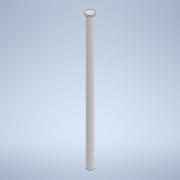
# Autodesk Inventor part: q1
Saved by Autodesk Inventor 2022 (Build 260153000, 153)
## iProperties
Created: 2023-05-29
Part Number: q1
Material: Ogólny
Document SubType Name: Modeling
Designer: nosal
Density: 1 g/cm^3
Appearance: Domyślna
Author: nosal
## iProperties of the stored document q1_Drukowanie 3D.ipt
Created: 2023-05-29
Part Number: q1_Drukowanie 3D
Material: Ogólny
Document SubType Name: Modeling
Designer: nosal
Density: 1 g/cm^3
Appearance: Domyślna
Author: nosal
Autodesk Inventor part; units mm, degrees
ref_plane "YZ Plane" through (0, 0, 0) normal (1, 0, 0) x (0, 1, 0)
ref_plane "XZ Plane" through (0, 0, 0) normal (0, 1, 0) x (-1, 0, 0)
ref_plane "XY Plane" through (0, 0, 0) normal (0, 0, 1) x (1, 0, 0)
sketch "Szkic1" plane through (0, 0, 0) normal (0, 0, 1) x (1, 0, 0)
  line L0 (0, 0) -> (-4, 0)
  line L1 (-4, 0) -> (-4, 175)
  line L2 (-4, 175) -> (0, 175)
  line L3 (0, 175) -> (0, 0)
  line L4 (-4, 175) -> (-5, 175)
  line L5 (-5, 175) -> (-5, 177)
  line L6 (-5, 177) -> (0, 177)
  line L7 (0, 177) -> (0, 175)
  dimension "d0" = 175
  dimension "d1" = 4
  dimension "d14" = 1
  dimension "d15" = 2
  constraints: 16 end point, 4 perpendicular, 2 horizontal, 2 parallel
  measures "d0" distance of L0.end L1.end
  measures "d1" distance of L1.end L2.end
  measures "d14" distance of L1.end L4.end
  measures "d15" distance of L4.end L5.end
revolve "Obrót5" add sketch "Szkic1" angle 360 about axis through (0, 175, 0) along (0, -1, 0)
sketch "Szkic2" plane through (0, 0, 0) normal (0, -1, 0) x (1, 0, 0)
  circle A0 centre (0, 0) radius 1
  dimension "d17" = 2
  constraints: 1 centre point, 1 coincident
  measures "d17" diameter of A0
extrude "Wyciągnięcie proste1" cut sketch "Szkic2" against normal blind 4
